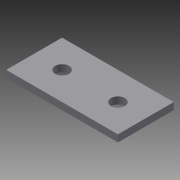
# Autodesk Inventor part: pickup arm gusset
Saved by Autodesk Inventor 2015 SP1 (Build 190203100, 203)
## iProperties
Created: 2015-01-28
Part Number: pickup arm gusset
Material: Generic
Document SubType Name: Modeling
Designer: Admin
Density: 1 g/cm^3
Appearance: Default
Author: Admin
Autodesk Inventor part; units mm, degrees
ref_plane "YZ Plane" through (0, 0, 0) normal (1, 0, 0) x (0, 1, 0)
ref_plane "XZ Plane" through (0, 0, 0) normal (0, 1, 0) x (-1, 0, 0)
ref_plane "XY Plane" through (0, 0, 0) normal (0, 0, 1) x (1, 0, 0)
sketch "Sketch1" plane through (0, 0, 0) normal (0, 1, 0) x (-1, 0, 0)
  line L0 (0, 0) -> (-76.2, 0)
  line L1 (-76.2, 0) -> (-76.2, 25.4)
  line L2 (-76.2, 25.4) -> (0, 25.4)
  line L3 (0, 25.4) -> (0, 0)
  dimension "d0" = 76.2
  dimension "d1" = 25.4
  constraints: 8 end point, 2 parallel, 1 horizontal, 1 perpendicular
  measures "d0" distance of L1.end L2.end
  measures "d1" distance of L0.end L1.end
extrude "Extrusion1" add sketch "Sketch1" along normal blind 3.175
sketch "Sketch2" plane through (0, 3.175, 0) normal (0, 1, 0) x (1, 0, 0)
  line L0 (76.2, 0) -> (0, 0) projected
  line L1 (0, 0) -> (0, -25.4) projected
  line L2 (76.2, -25.4) -> (76.2, 0) projected
  point P0 (12.7, -12.7)
  point P1 (63.5, -12.7)
  dimension "d4" = 12.7
  dimension "d5" = 12.7
  dimension "d6" = 12.7
  dimension "d7" = 12.7
  measures "d4" distance from line of L1 point (12.7, -12.7)
  measures "d5" distance from line of L0 point (12.7, -12.7)
  measures "d6" distance from line of L0 point (63.5, -12.7)
  measures "d7" distance from line of L2 point (63.5, -12.7)
hole "Hole1" at (12.7, 3.175, 12.7) at (63.5, 3.175, 12.7) direction (0, -1, 0) diameter 6.35 end through all
body "Solid1"
